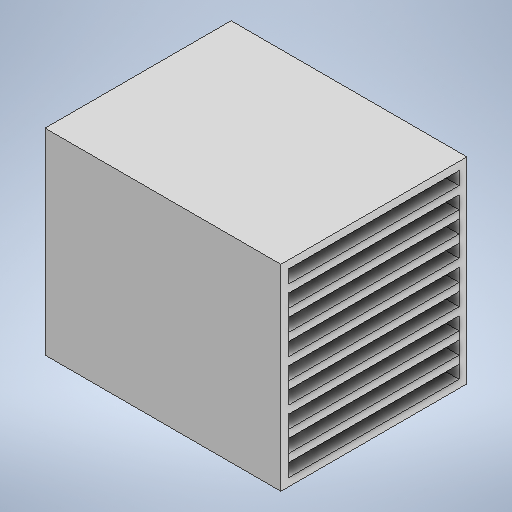
# Autodesk Inventor part: stack
Saved by Autodesk Inventor 2025.1 (Build 291241020, 241B)
## iProperties
Created: 2024-11-21
Part Number: stack
Material: Generic
Document SubType Name: Modeling
Designer: User
Density: 1 g/cm^3
Appearance: Default
Author: User
Autodesk Inventor part; units mm, degrees
ref_plane "YZ Plane" through (0, 0, 0) normal (1, 0, 0) x (0, 1, 0)
ref_plane "XZ Plane" through (0, 0, 0) normal (0, 1, 0) x (-1, 0, 0)
ref_plane "XY Plane" through (0, 0, 0) normal (0, 0, 1) x (1, 0, 0)
sketch "Sketch1" plane through (0, 0, 0) normal (0, 0, 1) x (1, 0, 0)
  line L0 (0, 0) -> (90, 0)
  line L1 (90, 0) -> (90, 3)
  line L2 (90, 3) -> (0, 3)
  line L3 (0, 3) -> (0, 0)
  line L4 (0, 8) -> (90, 8)
  line L5 (90, 8) -> (90, 11)
  line L6 (90, 11) -> (0, 11)
  line L7 (0, 11) -> (0, 8)
  line L8 (0, 16) -> (90, 16)
  line L9 (90, 16) -> (90, 19)
  line L10 (90, 19) -> (0, 19)
  line L11 (0, 19) -> (0, 16)
  line L12 (0, 24) -> (90, 24)
  line L13 (90, 24) -> (90, 27)
  line L14 (90, 27) -> (0, 27)
  line L15 (0, 27) -> (0, 24)
  line L16 (0, 32) -> (90, 32)
  line L17 (90, 32) -> (90, 35)
  line L18 (90, 35) -> (0, 35)
  line L19 (0, 35) -> (0, 32)
  line L20 (0, 40) -> (90, 40)
  line L21 (90, 40) -> (90, 43)
  line L22 (90, 43) -> (0, 43)
  line L23 (0, 43) -> (0, 40)
  line L24 (0, 48) -> (90, 48)
  line L25 (90, 48) -> (90, 51)
  line L26 (90, 51) -> (0, 51)
  line L27 (0, 51) -> (0, 48)
  line L28 (0.0005, 56) -> (90.0005, 56)
  line L29 (90.0005, 56) -> (90.0005, 59)
  line L30 (90.0005, 59) -> (0.0005, 59)
  line L31 (0.0005, 59) -> (0.0005, 56)
  line L32 (0, 64) -> (90, 64)
  line L33 (90, 64) -> (90, 67)
  line L34 (90, 67) -> (0, 67)
  line L35 (0, 67) -> (0, 64)
  line L36 (0, 72) -> (90, 72)
  line L37 (90, 72) -> (90, 75)
  line L38 (90, 75) -> (0, 75)
  line L39 (0, 75) -> (0, 72)
  line L40 (0, 75) -> (90, 75)
  line L41 (90, 75) -> (90, 0)
  line L42 (90, 0) -> (0, 0)
  line L43 (0, 0) -> (0, 75)
  dimension "d0" = 3
  dimension "d1" = 90
  dimension "d2" = 3
  dimension "d3" = 90
  dimension "d4" = 3
  dimension "d5" = 90
  dimension "d6" = 3
  dimension "d7" = 90
  dimension "d8" = 3
  dimension "d9" = 90
  dimension "d10" = 3
  dimension "d11" = 90
  dimension "d12" = 3
  dimension "d13" = 90
  dimension "d14" = 3
  dimension "d15" = 90
  dimension "d16" = 3
  dimension "d17" = 90
  dimension "d18" = 3
  dimension "d19" = 90
  dimension "d20" = 5
  dimension "d21" = 5
  dimension "d22" = 5
  dimension "d23" = 5
  dimension "d24" = 5
  dimension "d25" = 5
  dimension "d26" = 5
  dimension "d27" = 5
  dimension "d28" = 5
  constraints: 88 end point, 22 parallel, 11 horizontal, 11 perpendicular
  measures "d0" distance of L2.end L0.start
  measures "d1" distance of L0.start L0.end
  measures "d2" distance of L6.end L4.start
  measures "d3" distance of L4.start L4.end
  measures "d4" distance of L10.end L8.start
  measures "d5" distance of L8.start L8.end
  measures "d6" distance of L14.end L12.start
  measures "d7" distance of L12.start L12.end
  measures "d8" distance of L18.end L16.start
  measures "d9" distance of L16.start L16.end
  measures "d10" distance of L23.start L23.end
  measures "d11" distance of L23.end L20.end
  measures "d12" distance of L27.start L27.end
  measures "d13" distance of L27.end L24.end
  measures "d14" distance of L31.start L31.end
  measures "d15" distance of L31.end L28.end
  measures "d16" distance of L35.start L35.end
  measures "d17" distance of L35.end L32.end
  measures "d18" distance of L39.start L39.end
  measures "d19" distance of L39.end L36.end
  measures "d20" distance between parallel lines of L34 L36
  measures "d21" distance between parallel lines of L30 L32
  measures "d22" distance between parallel lines of L26 L28
  measures "d23" distance between parallel lines of L18 L20
  measures "d24" distance between parallel lines of L22 L24
  measures "d25" distance between parallel lines of L2 L4
  measures "d26" distance between parallel lines of L6 L8
  measures "d27" distance between parallel lines of L10 L12
  measures "d28" distance between parallel lines of L14 L16
extrude "Extrusion1" add sketch "Sketch1" against normal blind 65 contours L3 L2 L1 L0 | L7 L6 L5 L4 | L11 L10 L9 L8 | L15 L14 L13 L12 | L19 L18 L17 L16 | L23 L22 L21 L20 | L27 L26 L25 L24 | L31 L30 L29 L28 | L35 L34 L33 L32 | L39 L38 L37 L36
sketch "Sketch2" plane through (0, 0, 0) normal (0, 0, 1) x (1, 0, 0)
  point P0 (0, 0)
sketch "Sketch3" plane through (0, 0, 0) normal (0, 0, 1) x (1, 0, 0)
  line L0 (0, 72) -> (0, 75) projected
  line L1 (90, 0) -> (0, 0)
  line L2 (0, 0) -> (0, 75)
  line L3 (0, 75) -> (90, 75)
  line L4 (90, 75) -> (90, 0)
  line L5 (0, 75) -> (90, 75)
  line L6 (90, 75) -> (90, 95)
  line L7 (90, 95) -> (0, 95)
  line L8 (0, 95) -> (0, 75)
  line L9 (0, 0) -> (90, 0)
  line L10 (90, 0) -> (90, -20)
  line L11 (90, -20) -> (0, -20)
  line L12 (0, -20) -> (0, 0)
  point P0 (0, 0)
  dimension "d35" = 20
  dimension "d36" = 90
  dimension "d37" = 20
  dimension "d38" = 90
  constraints: 24 end point, 6 parallel, 3 horizontal, 3 perpendicular
  measures "d35" distance of L5.end L6.end
  measures "d36" distance of L6.end L7.end
  measures "d37" distance of L9.end L10.end
  measures "d38" distance of L10.end L11.end
extrude "Extrusion2" add sketch "Sketch3" along normal blind 3 contours L0 L3 L4 L1 L2
sketch "Sketch4" plane through (0, 0, -65) normal (0, -1, 0) x (1, 0, 0)
  point P0 (0, 65)
sketch "Sketch5" plane through (0, 0, -65) normal (0, 0, -1) x (-1, 0, 0)
  line L0 (-90, 75) -> (0, 75) projected
  line L1 (-90, 75) -> (0, 75)
  line L2 (0, 75) -> (0, 0)
  line L3 (0, 0) -> (-90, 0)
  line L4 (-90, 0) -> (-90, 75)
  constraints: 8 end point, 2 parallel, 1 horizontal, 1 perpendicular
extrude "Extrusion3" add sketch "Sketch5" along normal blind 3
body "Solid1"
